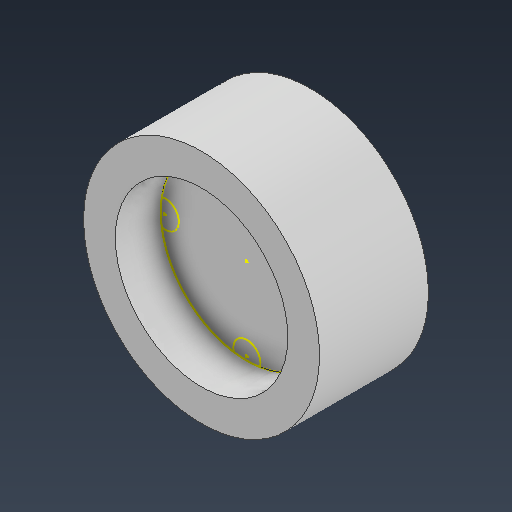
# Autodesk Inventor part: вт2
Saved by Autodesk Inventor 2025 (Build 290162000, 162)
## iProperties
Created: 2025-03-14
Part Number: вт2
Material: Типовые
Document SubType Name: Modeling
Designer: GameHD
Density: 1 g/cm^3
Appearance: По умолчанию
Author: GameHD
Autodesk Inventor part; units mm, degrees
ref_plane "YZ Plane" through (0, 0, 0) normal (1, 0, 0) x (0, 1, 0)
ref_plane "XZ Plane" through (0, 0, 0) normal (0, 1, 0) x (-1, 0, 0)
ref_plane "XY Plane" through (0, 0, 0) normal (0, 0, 1) x (1, 0, 0)
sketch "Эскиз1" plane through (0, 0, 0) normal (0, 0, 1) x (1, 0, 0)
  circle A0 centre (0, 0) radius 13
  circle A1 centre (0, 9) radius 1.5
  circle A2 centre (-9, 0) radius 1.5
  circle A3 centre (0, -9) radius 1.5
  circle A4 centre (9, 0) radius 1.5
  dimension "d0" = 26
  dimension "d1" = 3
  dimension "d2" = 9
  dimension "d5" = 360
  constraints: 5 centre point, 1 coincident, 9 other
  measures "d0" diameter of A0
  measures "d1" diameter of A1
  measures "d2" distance of point (0, 0) A1.centre
extrude "Выдавливание1" add sketch "Эскиз1" along normal blind 7
sketch "Эскиз2" plane through (0, 0, 7) normal (0, 0, 1) x (1, 0, 0)
  circle A0 centre (0, 0) radius 13 projected
  circle A1 centre (9, 0) radius 1.5 projected
  circle A2 centre (0, -9) radius 1.5 projected
  circle A3 centre (-9, 0) radius 1.5 projected
  circle A4 centre (0, 9) radius 1.5 projected
  circle A5 centre (0, 0) radius 9.5
  dimension "d9" = 19
  constraints: 2 coincident, 1 centre point
  measures "d9" diameter of A5
extrude "Выдавливание2" add sketch "Эскиз2" along normal blind 5 contours A0 | A1 A5 | A5 A4 | A2 A5 | A5 A3 picked at (9.8174, -0.2697) picked at (-0.0593, 9.8216) picked at (0.0593, -9.8216) picked at (-9.8216, 0.0593)
sketch "Эскиз3" plane through (0, 0, 7) normal (0, 0, 1) x (1, 0, 0)
  arc A0 (-1.4487, 9.3889) -> (-9.3889, 1.4487) centre (0, 0) ccw projected
  arc A1 (-9.3889, -1.4487) -> (-9.3889, 1.4487) centre (-9, 0) ccw projected
  arc A2 (-9.3889, -1.4487) -> (-1.4487, -9.3889) centre (0, 0) ccw projected
  arc A3 (1.4487, -9.3889) -> (-1.4487, -9.3889) centre (0, -9) ccw projected
  arc A4 (1.4487, -9.3889) -> (9.3889, -1.4487) centre (0, 0) ccw projected
  arc A5 (9.3889, 1.4487) -> (9.3889, -1.4487) centre (9, 0) ccw projected
  arc A6 (9.3889, 1.4487) -> (1.4487, 9.3889) centre (0, 0) ccw projected
  arc A7 (-1.4487, 9.3889) -> (1.4487, 9.3889) centre (0, 9) ccw projected
  arc A8 (1.4487, 9.3889) -> (-1.4487, 9.3889) centre (0, 0) ccw projected
  circle A9 centre (0, 0) radius 9.5 projected
  arc A10 (9.3889, -1.4487) -> (9.3889, 1.4487) centre (0, 0) ccw projected
  arc A11 (1.4487, -9.3889) -> (9.3889, -1.4487) centre (0, 0) ccw projected
  arc A12 (-1.4487, -9.3889) -> (1.4487, -9.3889) centre (0, 0) ccw projected
  arc A13 (-9.3889, -1.4487) -> (-1.4487, -9.3889) centre (0, 0) ccw projected
  arc A14 (-9.3889, 1.4487) -> (-9.3889, -1.4487) centre (0, 0) ccw projected
  arc A15 (-1.4487, 9.3889) -> (-9.3889, 1.4487) centre (0, 0) ccw projected
  arc A16 (1.4487, 9.3889) -> (-1.4487, 9.3889) centre (0, 0) ccw projected
  arc A17 (9.3889, 1.4487) -> (1.4487, 9.3889) centre (0, 0) ccw projected
  point P0 (-1.4487, -9.3889)
  point P1 (1.4487, -9.3889)
  point P2 (9.3889, -1.4487)
  point P3 (9.3889, 1.4487)
  point P4 (-9.3889, 1.4487)
  point P5 (-9.3889, -1.4487)
extrude "Выдавливание3" add sketch "Эскиз3" against normal blind 0.1 contours A8 A7 | A1 A9 | A9 A5 | A3 A9
